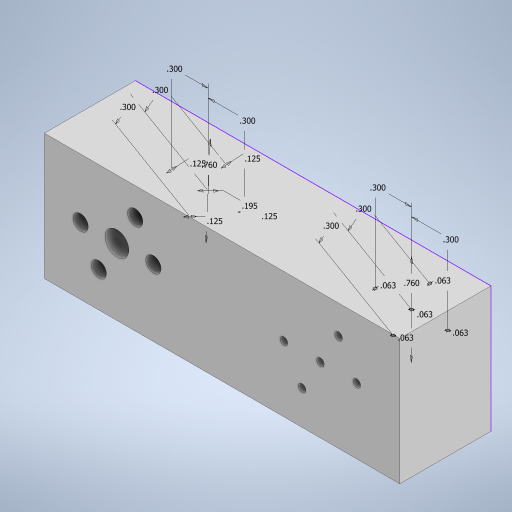
# Autodesk Inventor part: C.Crank Connect Shaft Cutting Jig
Saved by Autodesk Inventor 2023 (Build 270158000, 158)
## iProperties
Created: 2022-10-29
Part Number: C.Crank Connect Shaft Cutting Jig
Material: Generic
Document SubType Name: Modeling
Designer: tommy
Density: 1 g/cm^3
Appearance: Default
Author: tommy
Autodesk Inventor part; units mm, degrees
ref_plane "YZ Plane" through (0, 0, 0) normal (1, 0, 0) x (0, 1, 0)
ref_plane "XZ Plane" through (0, 0, 0) normal (0, 1, 0) x (-1, 0, 0)
ref_plane "XY Plane" through (0, 0, 0) normal (0, 0, 1) x (1, 0, 0)
sketch "Sketch1" plane through (0, 0, 0) normal (0, 0, 1) x (1, 0, 0)
  circle A0 centre (49.887, 0) radius 0.7937
  circle A1 centre (34.647, 0) radius 0.7937
  circle A2 centre (42.267, 0) radius 9.525
  circle A3 centre (38.457, -6.5991) radius 0.7937
  circle A4 centre (46.077, 6.5991) radius 0.7937
  circle A5 centre (42.267, 0) radius 0.7937
  line L0 (-15.4509, 12.6033) -> (58.8878, 12.6033)
  line L1 (58.8878, 12.6033) -> (58.8878, -13.7292)
  line L2 (58.8878, -13.7292) -> (-15.4509, -13.7292)
  line L3 (-15.4509, -13.7292) -> (-15.4509, 12.6033)
  circle A6 centre (7.3609, 0.2473) radius 1.5875
  circle A7 centre (-7.8791, 0.2473) radius 1.5875
  circle A8 centre (-0.2591, 0.2473) radius 9.525
  circle A9 centre (3.5509, 6.8464) radius 1.5875
  circle A10 centre (-4.0691, -6.3518) radius 1.5875
  circle A11 centre (-0.2591, 0.2473) radius 2.4765
  circle A12 centre (42.267, 0) radius 9.652
  circle A13 centre (-0.2591, 0.2473) radius 9.652
  point P0 (37.5045, -8.2489)
  point P1 (47.0295, 8.2489)
  point P2 (-5.0216, -8.0016)
  point P3 (4.5034, 8.4962)
  dimension "d69" = 1.5875
  dimension "d70" = 1.5875
  dimension "d75" = 1.5875
  dimension "d76" = 1.5875
  dimension "d79" = 7.62
  dimension "d80" = 7.62
  dimension "d82" = 1.5875
  dimension "d83" = 7.62
  dimension "d84" = 7.62
  dimension "d85" = 3.175
  dimension "d86" = 3.175
  dimension "d87" = 3.175
  dimension "d88" = 3.175
  dimension "d89" = 7.62
  dimension "d90" = 7.62
  dimension "d91" = 4.953
  dimension "d92" = 7.62
  dimension "d93" = 7.62
  dimension "d95" = 19.304
  dimension "d96" = 19.304
  constraints: 12 centre point, 12 coincident, 8 end point, 2 parallel, 1 horizontal, 1 perpendicular, 6 other
  measures "d69" diameter of A1
  measures "d70" diameter of A0
  measures "d75" diameter of A4
  measures "d76" diameter of A3
  measures "d79" distance of A4.centre point (42.267, 0)
  measures "d80" distance of point (42.267, 0) A3.centre
  measures "d82" diameter of A5
  measures "d83" distance of point (42.267, 0) A0.centre
  measures "d84" distance of point (42.267, 0) A1.centre
  measures "d85" diameter of A7
  measures "d86" diameter of A6
  measures "d87" diameter of A9
  measures "d88" diameter of A10
  measures "d89" distance of A9.centre point (-0.259, 0.247)
  measures "d90" distance of point (-0.259, 0.247) A10.centre
  measures "d91" diameter of A11
  measures "d92" distance of point (-0.259, 0.247) A6.centre
  measures "d93" distance of point (-0.259, 0.247) A7.centre
  measures "d95" diameter of A12
  measures "d96" diameter of A13
extrude "Extrusion14" add sketch "Sketch1" along normal blind 19.05 contours A2 | L0 L1 L2 L3 | A8 | A12 | A13
extrude "Extrusion15" cut sketch "Sketch1" along normal blind 11.938 contours A0 | A1 | A2 | A3 | A4 | A5 | A6 | A7 | A8 | A9 | A10 | A11 | A12 | A13
body "Solid5"
